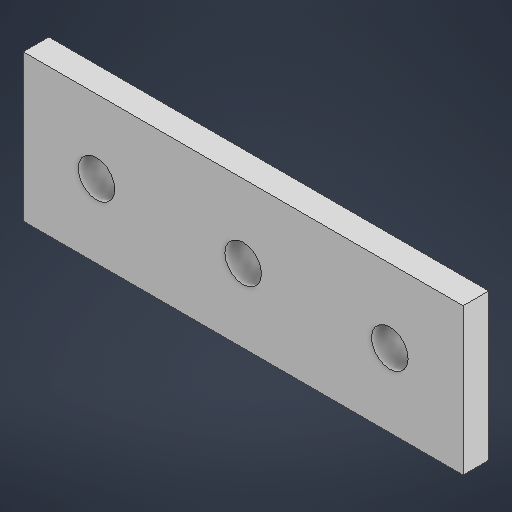
# Autodesk Inventor part: 2020 3 Bracket
Saved by Autodesk Inventor 2026 (Build 300175050, 175E)
## iProperties
Created: 2025-11-17
Part Number: 2020 3 Bracket
Material: Generic
Document SubType Name: Modeling
Designer: habbo
Density: 1 g/cm^3
Appearance: Default
Author: habbo
Autodesk Inventor part; units mm, degrees
ref_plane "YZ Plane" through (0, 0, 0) normal (1, 0, 0) x (0, 1, 0)
ref_plane "XZ Plane" through (0, 0, 0) normal (0, 1, 0) x (-1, 0, 0)
ref_plane "XY Plane" through (0, 0, 0) normal (0, 0, 1) x (1, 0, 0)
sketch "Sketch1" plane through (0, 0, 0) normal (0, 0, 1) x (1, 0, 0)
  line L0 (-30, -10) -> (30, -10)
  line L1 (30, -10) -> (30, 10)
  line L2 (30, 10) -> (-30, 10)
  line L3 (-30, 10) -> (-30, -10)
  line L4 (-30, -10) -> (30, 10) construction
  line L5 (30, -10) -> (-30, 10) construction
  circle A0 centre (-20, 0) radius 2.5
  circle A1 centre (0, 0) radius 2.5
  circle A2 centre (20, 0) radius 2.5
  point P0 (0, 0)
  dimension "d0" = 60
  dimension "d1" = 20
  dimension "d2" = 5
  dimension "d3" = 5
  dimension "d4" = 20
  dimension "d5" = 10
  dimension "d6" = 5
  dimension "d7" = 20
  dimension "d8" = 10
  constraints: 12 end point, 3 centre point, 2 midpoint, 2 parallel, 1 horizontal, 1 perpendicular
  measures "d0" distance of L2.end L1.end
  measures "d1" distance of L1.end L0.end
  measures "d2" diameter of A0
  measures "d3" diameter of A1
  measures "d4" distance of A1.centre A0.centre
  measures "d5" distance from line of L3 A0.centre
  measures "d6" diameter of A2
  measures "d7" distance of A2.centre point (0, 0)
  measures "d8" distance from line of L0 A0.centre
extrude "Extrusion1" add sketch "Sketch1" along normal mid plane 3.5
body "Solid1"
